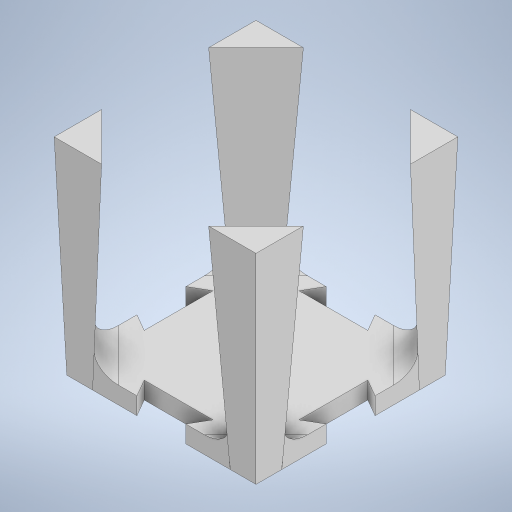
# Autodesk Inventor part: Duck_Holder
Saved by Autodesk Inventor 2024.4 (Build 284460000, 460)
## iProperties
Created: 2025-10-23
Part Number: Duck_Holder
Material: Generic
Document SubType Name: Modeling
Designer: Shane
Density: 1 g/cm^3
Appearance: Default
Author: Shane
Autodesk Inventor part; units mm, degrees
ref_plane "YZ Plane" through (0, 0, 0) normal (1, 0, 0) x (0, 1, 0)
ref_plane "XZ Plane" through (0, 0, 0) normal (0, 1, 0) x (-1, 0, 0)
ref_plane "XY Plane" through (0, 0, 0) normal (0, 0, 1) x (1, 0, 0)
sketch "Sketch1" plane through (0, 0, 0) normal (0, 1, 0) x (-1, 0, 0)
  line L0 (0, 0) -> (55, 0)
  line L1 (55, 0) -> (55, -55)
  line L2 (55, -55) -> (0, -55)
  line L3 (0, -55) -> (0, 0)
  line L4 (55, -27.5) -> (0, -27.5) construction
  line L5 (27.5, -55) -> (27.5, 0) construction
  line L6 (20.3868, -55) -> (34.6132, -55)
  line L7 (34.6842, -50) -> (21.2609, -50)
  line L8 (50, -17.5) -> (50, -33.6438)
  line L9 (55, -34.6132) -> (55, -20.3868)
  line L10 (5, -18.3051) -> (5, -36.8563)
  line L11 (0, -34.6132) -> (0, -20.3868)
  line L12 (20.3868, 0) -> (34.6132, 0)
  line L13 (37.7365, -5) -> (17.5, -5)
  line L14 (55, -34.6132) -> (50, -37.5)
  line L15 (50, -37.5) -> (50, -33.6438)
  line L16 (55, -20.3868) -> (50, -17.5)
  line L17 (34.6842, -50) -> (37.5, -50)
  line L18 (37.5, -50) -> (34.6132, -55)
  line L19 (21.2609, -50) -> (17.5, -50)
  line L20 (17.5, -50) -> (20.3868, -55)
  line L21 (0, -34.6132) -> (5, -37.5)
  line L22 (5, -37.5) -> (5, -36.8563)
  line L23 (0, -20.3868) -> (5, -17.5)
  line L24 (5, -17.5) -> (5, -18.3051)
  line L25 (20.3868, 0) -> (17.5, -5)
  line L26 (34.6132, 0) -> (37.5, -5)
  line L27 (37.5, -5) -> (37.7365, -5)
  line L28 (55, -47.5) -> (47.5, -55)
  line L29 (55, -7.5) -> (47.5, 0)
  line L30 (7.5, -55) -> (0, -47.5)
  line L31 (7.5, 0) -> (0, -7.5)
  line L32 (55, 0) -> (0, 0)
  line L33 (0, 0) -> (0, -55)
  line L34 (0, -55) -> (55, -55)
  line L35 (55, -55) -> (55, 0)
  dimension "d0" = 55
  dimension "d1" = 55
  dimension "d4" = 5
  dimension "d5" = 5
  dimension "d6" = 60
  dimension "d9" = 60
  dimension "d10" = 60
  dimension "d13" = 20
  dimension "d14" = 10
  dimension "d15" = 60
  dimension "d16" = 5
  dimension "d18" = 60
  dimension "d19" = 5
  dimension "d20" = 20
  dimension "d21" = 10
  dimension "d22" = 10
  dimension "d23" = 20
  dimension "d24" = 20
  dimension "d25" = 10
  dimension "d26" = 7.5
  dimension "d27" = 7.5
  dimension "d28" = 7.5
  dimension "d29" = 7.5
  dimension "d30" = 7.5
  dimension "d31" = 7.5
  constraints: 72 end point, 15 point on line, 8 parallel, 7 perpendicular, 5 horizontal, 4 midpoint, 1 collinear, 1 vertical
  measures "d0" distance of L0.end L1.end
  measures "d1" distance of L1.end L2.end
  measures "d4" distance between parallel lines of L2 L7
  measures "d5" distance between parallel lines of L3 L10
  measures "d6" angle of L12 L26
  measures "d9" angle of L1 L14
  measures "d10" angle of L3 L21
  measures "d13" distance of L14.end L8.start
  measures "d14" distance from line of L4 L8.start
  measures "d15" angle of L1 L16
  measures "d16" distance between parallel lines of L1 L15
  measures "d18" angle of L0 L25
  measures "d19" distance between parallel lines of L0 L13
  measures "d20" distance of L13.end L26.end
  measures "d21" distance from line of L5 L13.end
  measures "d22" distance from line of L4 L23.end
  measures "d23" distance of L21.end L23.end
  measures "d24" distance of L17.end L19.end
  measures "d25" distance from line of L5 L19.end
  measures "d26" distance of L1.end L28.end
  measures "d27" distance of L1.end L28.start
  measures "d28" distance of L0.end L29.end
  measures "d29" distance of L29.start L0.end
  measures "d30" distance of L2.end L30.end
  measures "d31" distance of L0.start L31.end
extrude "Extrusion1" add sketch "Sketch1" along normal blind 5 contours L0 L25 L13 L26 L29 L1 L16 L8 L15 L14 L28 L2 L18 L17 L7 L19 L20 L30 L3 L21 L22 L10 L24 L23 L31
extrude "Extrusion2" add sketch "Sketch1" along normal blind 60 draft 1.75 contours L0 L31 L3 | L0 L1 L29 | L30 L2 L3 | L1 L2 L28
fillet "Fillet1" radius 5 4 edges at (-3.858, 5, -51.142) (-3.858, 5, -3.858) (-51.142, 5, -51.142) (-51.142, 5, -3.858)
equation "\"d0\" = side_length"
equation "\"d1\" = side_length"
equation "\"d4\" = dovetail_depth"
equation "\"d5\" = dovetail_depth"
equation "\"d13\" = dovetail_max_length"
equation "\"d14\" = 0.5 * dovetail_max_length"
equation "\"d16\" = dovetail_depth"
equation "\"d19\" = dovetail_depth"
equation "\"d20\" = dovetail_max_length"
equation "\"d21\" = 0.5 * dovetail_max_length"
equation "\"d22\" = 0.5 * dovetail_max_length"
equation "\"d23\" = dovetail_max_length"
equation "\"d24\" = dovetail_max_length"
equation "\"d25\" = 0.5 * dovetail_max_length"
equation "\"d26\" = claw_wall_side_length"
equation "\"d27\" = claw_wall_side_length"
equation "\"d28\" = claw_wall_side_length"
equation "\"d29\" = claw_wall_side_length"
equation "\"d30\" = claw_wall_side_length"
equation "\"d31\" = claw_wall_side_length"
equation "\"side_length\" = 55"
equation "\"dovetail_depth\" = 5"
equation "\"dovetail_max_length\" = 20"
equation "\"claw_wall_side_length\" = 7.5"
equation "\"band_notch_height\" = 45"
body "Solid1"
